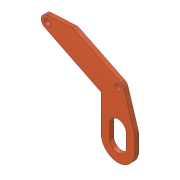
# Autodesk Inventor part: COXA_YAW_SUPPORT-LINK_BACK
Saved by Autodesk Inventor 2019.4 (Build 234330000, 330)
## iProperties
Created: 2019-10-21
Part Number: COXA_YAW_SUPPORT-LINK_BACK
Material: 一般
Document SubType Name: Modeling
Designer: y6tada
Density: 1 g/cm^3
Appearance: 滑らか - 淡いオレンジ
Author: y6tada
Autodesk Inventor part; units mm, degrees
ref_plane "YZ Plane" through (0, 0, 0) normal (1, 0, 0) x (0, 1, 0)
ref_plane "XZ Plane" through (0, 0, 0) normal (0, 1, 0) x (-1, 0, 0)
ref_plane "XY Plane" through (0, 0, 0) normal (0, 0, 1) x (1, 0, 0)
sketch "スケッチ1" plane through (0, 0, 0) normal (0, 0, 1) x (1, 0, 0)
  line L0 (0, 0) -> (0, -20) construction
  line L1 (0, -20) -> (-33.541, 10) construction
  line L2 (-33.541, 10) -> (0, 0) construction
  arc A0 (-33.6899, 12.9963) -> (-34.8652, 7.3081) centre (-33.541, 10) ccw
  arc A1 (2.8673, 0.8824) -> (1.3242, 2.6919) centre (0, 0) ccw
  arc A2 (-8, -23) -> (8, -23) centre (0, -23) ccw
  arc A3 (4, -17) -> (-4, -17) centre (0, -17) ccw
  arc A4 (-4, -23) -> (4, -23) centre (0, -23) ccw
  line L3 (-4, -17) -> (-4, -23)
  line L4 (4, -17) -> (4, -23)
  line L5 (0, -23) -> (0, -17) construction
  line L6 (2.8673, 0.8824) -> (7.6462, -14.6471)
  line L7 (8, -17) -> (8, -23)
  arc A5 (8, -17) -> (7.6462, -14.6471) centre (0, -17) ccw
  line L8 (-33.6899, 12.9963) -> (-21.6899, 13.5926)
  line L9 (-20.2168, 13.2882) -> (1.3242, 2.6919)
  arc A6 (-20.2168, 13.2882) -> (-21.6899, 13.5926) centre (-21.541, 10.5963) ccw
  line L10 (-33.541, 10) -> (-21.541, 10.5963) construction
  line L11 (-8, -23) -> (-8, -5.9073)
  line L12 (-8, -5.9073) -> (-34.8652, 7.3081)
  dimension "d0" = 20
  dimension "d1" = 45
  dimension "d2" = 35
  dimension "d3" = 3
  dimension "d13" = 6
  dimension "d14" = 4
  dimension "d15" = 8
  dimension "d17" = 3
  dimension "d18" = 4
  dimension "d20" = 12
  constraints: 26 end point, 16 point on circle, 14 tangent, 7 centre point, 6 coincident, 3 point on line, 3 vertical, 2 concentric, 2 equal radius, 1 midpoint, 1 parallel
  measures "d0" distance of L0.end L0.start
  measures "d1" distance of L0.end L1.end
  measures "d2" distance of L1.end L0.start
  measures "d3" radius of A0
  measures "d13" distance of L5.start L5.end
  measures "d14" radius of A3
  measures "d15" radius of A2
  measures "d17" radius of A6
  measures "d18" distance from line of L10.end L2
  measures "d20" horizontal distance of L10.start L10.end
extrude "押し出し1" add sketch "スケッチ1" along normal blind 2
hole "穴1" at (-33.541, 10, 0) at (0, 0, 0) direction (0, 0, 1) diameter 3 end through all
